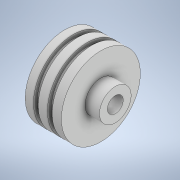
# Autodesk Inventor part: Part5
Saved by Autodesk Inventor 2021 (Build 250183000, 183)
## iProperties
Created: 2022-06-05
Part Number: Part5
Material: Generic
Document SubType Name: Modeling
Designer: Bhargav Malasani
Density: 1 g/cm^3
Appearance: Default
Author: Bhargav Malasani
Autodesk Inventor part; units mm, degrees
ref_plane "YZ Plane" through (0, 0, 0) normal (1, 0, 0) x (0, 1, 0)
ref_plane "XZ Plane" through (0, 0, 0) normal (0, 1, 0) x (-1, 0, 0)
ref_plane "XY Plane" through (0, 0, 0) normal (0, 0, 1) x (1, 0, 0)
sketch "Sketch1" plane through (0, 0, 0) normal (0, 0, 1) x (1, 0, 0)
  line L0 (0, 0) -> (38.5, 0)
  line L1 (38.5, 6) -> (16, 6)
  line L2 (38.5, 12) -> (27.5, 12)
  line L3 (27.5, 12) -> (27.5, 30)
  line L4 (27.5, 30) -> (20.5, 30)
  line L5 (20.5, 30) -> (20.5, 27.2)
  line L6 (20.5, 27.2) -> (16.9, 27.2)
  line L7 (16.9, 27.2) -> (16.9, 30)
  line L8 (16.9, 30) -> (9.9, 30)
  line L9 (9.9, 30) -> (9.9, 27.2)
  line L10 (9.9, 27.2) -> (6.3, 27.2)
  line L11 (6.3, 27.2) -> (6.3, 30)
  line L12 (0, 0) -> (0, 30)
  line L13 (0, 30) -> (6.3, 30)
  line L14 (38.5, 6) -> (38.5, 12)
  line L15 (16, 6) -> (16, 12)
  line L16 (16, 12) -> (19, 12)
  line L17 (21, 14) -> (21, 17.5036)
  line L18 (0, 23) -> (18.751, 19.6937)
  line L19 (21, 17.5036) -> (21, 17.6189)
  line L20 (19.3473, 19.5885) -> (18.751, 19.6937)
  arc A0 (19, 12) -> (21, 14) centre (19, 14) ccw
  arc A1 (21, 17.6189) -> (19.3473, 19.5885) centre (19, 17.6189) ccw
  point P0 (21, 12)
  dimension "d0" = 38.5
  dimension "d1" = 22.5
  dimension "d2" = 38.5
  dimension "d3" = 6
  dimension "d4" = 11
  dimension "d5" = 7
  dimension "d6" = 2.8
  dimension "d7" = 3.6
  dimension "d8" = 7
  dimension "d9" = 2.8
  dimension "d10" = 3.6
  dimension "d12" = 12
  dimension "d13" = 30
  dimension "d14" = 27.5
  dimension "d15" = 21
  dimension "d16" = 23
  dimension "d17" = 10
  dimension "d18" = 2
  dimension "d19" = 2
  constraints: 42 end point, 9 point on line, 8 perpendicular, 4 horizontal, 4 point on circle, 4 tangent, 3 vertical, 2 centre point, 1 equal radius
  measures "d0" distance of L0.start L0.end
  measures "d1" distance of L1.start L1.end
  measures "d2" horizontal distance of L0.start L1.start
  measures "d3" distance between parallel lines of L0 L1
  measures "d4" distance of L2.start L2.end
  measures "d5" distance of L3.end L4.end
  measures "d6" distance of L4.end L5.end
  measures "d7" distance of L5.end L6.end
  measures "d8" distance of L7.end L8.end
  measures "d9" distance of L8.end L9.end
  measures "d10" distance of L9.end L10.end
  measures "d12" distance between parallel lines of L0 L2
  measures "d13" distance between parallel lines of L0 L4
  measures "d14" distance between parallel lines of L3 L12
  measures "d15" distance from line of L12 point (21, 12)
  measures "d16" distance of L0.start L18.start
  measures "d17" angle of L0 L18
  measures "d18" radius of A0
  measures "d19" distance from line of L18 A1.centre
revolve "Revolution1" add sketch "Sketch1" angle 360 about axis through (0, 0, 0) along (1, 0, 0)
equation "\"d2\" = d0"
body "Solid1"
